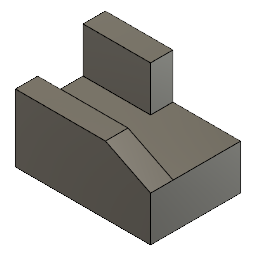
3DD5 (Autodesk Fusion 360 design; units mm, degrees)
Autodesk Fusion 360 part; units mm, degrees
sketch "Sketch1" plane through (0, 0, 0) normal (0, 1, 0) x (1, 0, 0)
  line L0 (0, 0) -> (60, 0)
  line L1 (60, 0) -> (60, -40)
  line L2 (60, -40) -> (0, -40)
  line L3 (0, -40) -> (0, 0)
  dimension "d1" = 60
  dimension "d2" = 40
  measures "d1" distance of L0.start
  measures "d2" distance of L0.start
extrude "Extrude1" add sketch "Sketch1" along normal blind 20
sketch "Sketch2" plane through (0, 20, 0) normal (0, 1, 0) x (-1, 0, 0)
  line L0 (0, 40) -> (-60, 40)
  line L1 (-60, 40) -> (-60, 0)
  line L2 (-60, 0) -> (0, 0)
  line L3 (0, 0) -> (0, 40)
  line L4 (0, 0) -> (-30, 0)
  line L5 (-30, 0) -> (-30, 10)
  line L6 (-30, 10) -> (0, 10)
  line L7 (0, 10) -> (0, 0)
  dimension "d5" = 30
  dimension "d6" = 10
  measures "d6" distance of L2.end
extrude "Extrude2" add sketch "Sketch2" along normal blind 20 contours L2 L3 L4 L5 L6 L7
sketch "Sketch3" plane through (0, 20, 0) normal (0, 1, 0) x (-1, 0, 0)
  line L0 (-30, 0) -> (-30, 10)
  line L1 (-30, 10) -> (0, 10)
  line L2 (0, 10) -> (0, 40)
  line L3 (0, 40) -> (-60, 40)
  line L4 (-60, 40) -> (-60, 0)
  line L5 (-60, 0) -> (-30, 0)
  line L6 (0, 30) -> (-60, 30)
  line L7 (-60, 30) -> (-60, 40)
  line L8 (-60, 40) -> (0, 40)
  line L9 (0, 40) -> (0, 30)
  dimension "d9" = 10
  measures "d9" distance of origin
extrude "Extrude3" add sketch "Sketch3" along normal blind 10 contours L2 L3 L4 L6 L7 L8 L9
sketch "Sketch4" plane through (0, 0, 30) normal (0, 0, -1) x (-1, 0, 0)
  line L0 (-60, 20) -> (0, 20)
  line L1 (0, 20) -> (0, 30)
  line L2 (0, 30) -> (-60, 30)
  line L3 (-60, 30) -> (-60, 20)
  line L4 (-60, 20) -> (-40, 30)
  line L5 (-60, 20) -> (-60, 30)
  line L6 (-40, 30) -> (-60, 30)
  dimension "d12" = 20
extrude "Extrude4" cut sketch "Sketch4" against normal blind 10 contours L2 L3 L4 L5 L6
